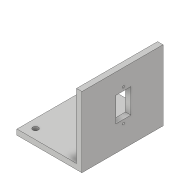
# Autodesk Inventor part: Part2
Saved by Autodesk Inventor 2019 (Build 230136000, 136)
## iProperties
Created: 2020-03-05
Part Number: Part2
Material: Generic
Document SubType Name: Modeling
Designer: Pranav naik
Density: 1 g/cm^3
Appearance: Default
Author: Pranav naik
Autodesk Inventor part; units mm, degrees
ref_plane "YZ Plane" through (0, 0, 0) normal (1, 0, 0) x (0, 1, 0)
ref_plane "XZ Plane" through (0, 0, 0) normal (0, 1, 0) x (-1, 0, 0)
ref_plane "XY Plane" through (0, 0, 0) normal (0, 0, 1) x (1, 0, 0)
sketch "Sketch1" plane through (0, 0, 0) normal (0, 0, 1) x (1, 0, 0)
  point P0 (0, 0)
sketch "Sketch2" plane through (0, 0, 0) normal (0, 0, 1) x (1, 0, 0)
  line L0 (0, 12.9308) -> (5, 12.9308)
  line L1 (5, 12.9308) -> (5, -47.0692)
  line L2 (0, -47.0692) -> (0, 12.9308)
  line L3 (0, -47.0692) -> (-55, -47.0692)
  line L4 (-55, -47.0692) -> (-55, -52.0692)
  line L5 (-55, -52.0692) -> (5, -52.0692)
  line L6 (5, -52.0692) -> (5, -47.0692)
  point P0 (0, 0)
  constraints: 14 end point, 3 parallel, 2 horizontal, 2 perpendicular
extrude "Extrusion1" add sketch "Sketch2" along normal blind 75
sketch "Sketch3" plane through (-55, -47.0692, 0) normal (0, 1, 0) x (1, 0, 0)
  circle A0 centre (8.2492, -7.6821) radius 2.5
  circle A1 centre (8.2492, -66.0616) radius 2.5
  point P0 (55, 0)
  dimension "d6" = 5
  dimension "d7" = 5
  constraints: 2 centre point
  measures "d6" diameter of A0
  measures "d7" diameter of A1
extrude "Extrusion2" cut sketch "Sketch3" against normal blind 75
sketch "Sketch4" plane through (5, -52.0692, 0) normal (1, 0, 0) x (0, 0, -1)
  line L0 (-43.5238, 46.3128) -> (-29.6738, 46.3128)
  line L1 (-29.6738, 46.3128) -> (-29.6738, 23.4735)
  line L2 (-29.6738, 23.4735) -> (-43.5238, 23.4735)
  line L3 (-43.5238, 23.4735) -> (-43.5238, 46.3128)
  point P0 (0, 52.0692)
  constraints: 8 end point, 2 parallel, 1 horizontal, 1 perpendicular
extrude "Extrusion3" cut sketch "Sketch4" against normal blind 75
sketch "Sketch5" plane through (5, -52.0692, 0) normal (1, 0, 0) x (0, 0, -1)
  line L0 (-43.5238, 46.3128) -> (-43.5238, 23.4735) projected
  line L1 (-43.5238, 46.3128) -> (-29.6738, 46.3128) projected
  line L2 (-43.5238, 46.3128) -> (-29.6738, 46.3128)
  line L3 (-43.5238, 46.3128) -> (-36.5988, 46.3128)
  circle A0 centre (-36.5988, 49.6128) radius 1
  circle A1 centre (-36.5988, 20.1735) radius 1
  point P0 (0, 52.0692)
  constraints: 4 end point, 2 centre point, 1 collinear, 1 midpoint
extrude "Extrusion4" cut sketch "Sketch5" against normal blind 75
body "Solid1"
